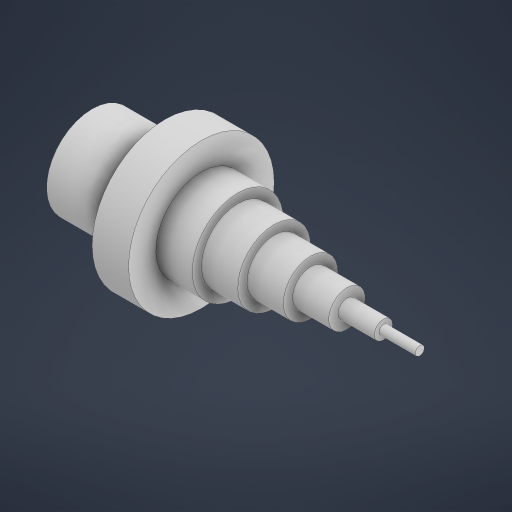
# Autodesk Inventor part: Część6
Saved by Autodesk Inventor 2023 (Build 270158000, 158)
## iProperties
Created: 2023-05-07
Part Number: Część6
Material: Ogólny
Document SubType Name: Modeling
Designer: Adam
Density: 1 g/cm^3
Appearance: Domyślna
Author: Adam
Autodesk Inventor part; units mm, degrees
ref_plane "YZ Plane" through (0, 0, 0) normal (1, 0, 0) x (0, 1, 0)
ref_plane "XZ Plane" through (0, 0, 0) normal (0, 1, 0) x (-1, 0, 0)
ref_plane "XY Plane" through (0, 0, 0) normal (0, 0, 1) x (1, 0, 0)
sketch "Szkic1" plane through (0, 0, 0) normal (0, 0, 1) x (1, 0, 0)
  line L0 (-16.6603, 0) -> (23.3397, 0)
  line L1 (23.3397, 0) -> (23.3397, 25)
  line L2 (23.3397, 25) -> (-16.6603, 25)
  line L3 (-16.6603, 25) -> (-16.6603, 0)
  line L4 (23.3397, 0) -> (43.3397, 0)
  line L5 (43.3397, 0) -> (43.3397, 40)
  line L6 (43.3397, 40) -> (23.3397, 40)
  line L7 (23.3397, 40) -> (23.3397, 0)
  line L8 (43.3397, 0) -> (63.3397, 0)
  line L9 (63.3397, 0) -> (63.3397, 25)
  line L10 (63.3397, 25) -> (43.3397, 25)
  line L11 (43.3397, 25) -> (43.3397, 0)
  line L12 (63.3397, 0) -> (83.3397, 0)
  line L13 (83.3397, 0) -> (83.3397, 20)
  line L14 (83.3397, 20) -> (63.3397, 20)
  line L15 (63.3397, 20) -> (63.3397, 0)
  line L16 (83.3397, 0) -> (103.3397, 0)
  line L17 (103.3397, 0) -> (103.3397, 15)
  line L18 (103.3397, 15) -> (83.3397, 15)
  line L19 (83.3397, 15) -> (83.3397, 0)
  line L20 (103.3397, 0) -> (123.3397, 0)
  line L21 (123.3397, 0) -> (123.3397, 10)
  line L22 (123.3397, 10) -> (103.3397, 10)
  line L23 (103.3397, 10) -> (103.3397, 0)
  line L24 (123.3397, 0) -> (143.3397, 0)
  line L25 (143.3397, 0) -> (143.3397, 5)
  line L26 (143.3397, 5) -> (123.3397, 5)
  line L27 (123.3397, 5) -> (123.3397, 0)
  line L28 (143.3397, 0) -> (163.3397, 0)
  line L29 (163.3397, 0) -> (163.3397, 2.5)
  line L30 (163.3397, 2.5) -> (143.3397, 2.5)
  line L31 (143.3397, 2.5) -> (143.3397, 0)
  point P0 (0, 0)
  dimension "d0" = 40
  dimension "d1" = 25
  dimension "d2" = 20
  dimension "d3" = 40
  dimension "d4" = 20
  dimension "d5" = 25
  dimension "d6" = 20
  dimension "d7" = 20
  dimension "d8" = 20
  dimension "d9" = 15
  dimension "d10" = 20
  dimension "d11" = 10
  dimension "d12" = 20
  dimension "d13" = 5
  dimension "d14" = 20
  dimension "d15" = 2.5
  constraints: 64 end point, 16 parallel, 8 horizontal, 8 perpendicular
  measures "d0" distance of L2.end L1.end
  measures "d1" distance of L1.end L0.end
  measures "d2" distance of L6.end L5.end
  measures "d3" distance of L5.end L4.end
  measures "d4" distance of L10.end L9.end
  measures "d5" distance of L9.end L8.end
  measures "d6" distance of L14.end L13.end
  measures "d7" distance of L13.end L12.end
  measures "d8" distance of L18.end L17.end
  measures "d9" distance of L17.end L16.end
  measures "d10" distance of L22.end L21.end
  measures "d11" distance of L21.end L20.end
  measures "d12" distance of L26.end L25.end
  measures "d13" distance of L25.end L24.end
  measures "d14" distance of L30.end L29.end
  measures "d15" distance of L29.end L28.end
revolve "Obrót1" add sketch "Szkic1" angle 360 about axis through (-16.6603, 0, 0) along (1, 0, 0)
sketch "Szkic2" plane through (-16.6603, 0, 0) normal (-1, 0, 0) x (0, 0, 1)
  point P0 (0, 0)
hole "Otwór1" at (-16.6603, 0, 0) direction (1, 0, 0) diameter 40 depth 40
